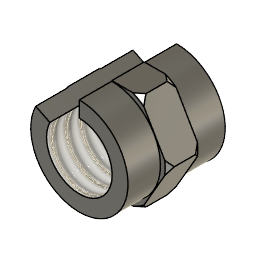
Packing Nut (Autodesk Fusion 360 design; units mm, degrees)
Autodesk Fusion 360 part; units mm, degrees
sketch "Sketch1" plane through (0, 0, 0) normal (0, 1, 0) x (1, 0, 0)
  line L0 (44.45, 0) -> (22.225, 38.4948)
  line L1 (22.225, 38.4948) -> (-22.225, 38.4948)
  line L2 (-22.225, 38.4948) -> (-44.45, 0)
  line L3 (-44.45, 0) -> (-22.225, -38.4948)
  line L4 (-22.225, -38.4948) -> (22.225, -38.4948)
  line L5 (22.225, -38.4948) -> (44.45, 0)
  dimension "d1" = 44.45
  measures "d1" distance of L0.start origin
extrude "Extrude1" add sketch "Sketch1" along normal blind 25.4
sketch "Sketch3" plane through (0, 0, 0) normal (0, 0, 1) x (1, 0, 0)
  line L0 (-41.8081, 0) -> (-44.45, 4.5759)
  line L1 (-44.45, 0) -> (-44.45, 25.4)
  line L2 (-44.45, 0) -> (-22.225, 0)
  line L3 (-44.45, 21.0433) -> (-41.9346, 25.4)
  line L4 (-44.45, 25.4) -> (-22.225, 25.4)
  dimension "d6" = 150
  dimension "d7" = 30
  constraint coincident L0.end L1
  constraint coincident L0.start L2
  constraint coincident L3.end L4
  constraint coincident L1 L3.start
  measures "d6" angle of L1 L3
  measures "d7" angle of L0 L1
revolve "Revolve1" cut sketch "Sketch3" angle 360 about axis through (0, 1.75, 0) along (0, 1, 0)
sketch "Sketch4" plane through (0, 0, 0) normal (0, -1, 0) x (1, 0, 0)
  arc A0 (25.1818, 33.3735) -> (16.3115, 38.4948) centre (0, 0) ccw
  line L0 (16.3115, 38.4948) -> (-16.3115, 38.4948)
  arc A1 (-16.3115, 38.4948) -> (-25.1818, 33.3735) centre (0, 0) ccw
  line L1 (-25.1818, 33.3735) -> (-41.4932, 5.1213)
  arc A2 (-41.4932, 5.1213) -> (-41.4932, -5.1213) centre (0, 0) ccw
  line L2 (-41.4932, -5.1213) -> (-25.1818, -33.3735)
  arc A3 (-25.1818, -33.3735) -> (-16.3115, -38.4948) centre (0, 0) ccw
  line L3 (-16.3115, -38.4948) -> (16.3115, -38.4948)
  arc A4 (16.3115, -38.4948) -> (25.1818, -33.3735) centre (0, 0) ccw
  line L4 (25.1818, -33.3735) -> (41.4932, -5.1213)
  arc A5 (41.4932, -5.1213) -> (41.4932, 5.1213) centre (0, 0) ccw
  line L5 (41.4932, 5.1213) -> (25.1818, 33.3735)
  circle A6 centre (0, 0) radius 38.1
  dimension "d9" = 76.2
  constraint coincident A0.centre A1.centre
  measures "d9" diameter of A6
extrude "Extrude2" add sketch "Sketch4" along normal blind 25.4 and the other way blind 50.8 contours A6
sketch "Sketch5" plane through (0, -25.4, 0) normal (0, -1, 0) x (1, 0, 0)
  circle A0 centre (0, 0) radius 38.1
  arc A1 (0, 38.1) -> (-34.0643, 17.0655) centre (0, 0) ccw
  line L0 (0, 39.0007) -> (0, 0)
  line L1 (0, 0) -> (-45.72, 0)
  arc A2 (0, 44.9703) -> (-40.4044, 19.7436) centre (0, 0) ccw
  line L2 (-40.4044, 19.7436) -> (0, 0)
  line L3 (0, 44.9703) -> (0, 0)
  constraint coincident A0 A1.start
  constraint coincident A0.centre A1.centre
  constraint vertical L0
  constraint perpendicular L0 L1
  constraint perpendicular L1 L3
extrude "Extrude3" cut sketch "Sketch5" against normal blind 76.2 contours A0 A1 L0 L2 L3 | A0 A1 L0 A2 L2 L3
hole "Hole1" at (0, -25.4, 0) direction (0, 1, 0) diameter 50.8 depth 76.2 tip angle 118
thread "Thread1" "ANSI Unified Screw Threads 2.25 2 1/4-4.5 UNC 2 1/4-4.5 UNC 3B" major diameter 57.15 minor diameter 51.374 pitch 5.6444 angle 60 resizes the face on face at (19.5442, 25.4, -16.2229)
scale "Scale4" factor 0.5 about (0, 50.8, 38.1) bodies 1
